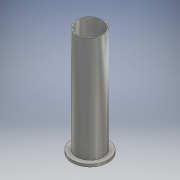
# Autodesk Inventor part: UR5 End to wrist
Saved by Autodesk Inventor 2016 (Build 200138000, 138)
## iProperties
Created: 2017-12-24
Part Number: UR5 End to wrist
Material: Aluminum 6061-AHC
Document SubType Name: Modeling
Designer: kornbot
Density: 2.7 g/cm^3
Appearance: Aluminum - Dark
Author: kornbot
Autodesk Inventor part; units mm, degrees
ref_plane "YZ Plane" through (0, 0, 0) normal (1, 0, 0) x (0, 1, 0)
ref_plane "XZ Plane" through (0, 0, 0) normal (0, 1, 0) x (-1, 0, 0)
ref_plane "XY Plane" through (0, 0, 0) normal (0, 0, 1) x (1, 0, 0)
sketch "Sketch1" plane through (0, 0, 0) normal (0, 0, 1) x (1, 0, 0)
  circle A0 centre (0, 0) radius 33.6825
  circle A1 centre (0, 0) radius 25
  dimension "d0" = 67.365
  dimension "d1" = 50
  constraints: 2 centre point, 2 coincident
  measures "d0" diameter of A0
  measures "d1" diameter of A1
extrude "Extrusion1" add sketch "Sketch1" along normal blind 5
sketch "Sketch2" plane through (0, 0, 5) normal (0, 0, 1) x (1, 0, 0)
  circle A0 centre (0, 0) radius 25
  circle A1 centre (0, 0) radius 23.5
  dimension "d4" = 47
  constraints: 2 centre point, 2 coincident
  measures "d4" diameter of A1
extrude "Extrusion2" add sketch "Sketch2" along normal blind 200
body "Solid1"
